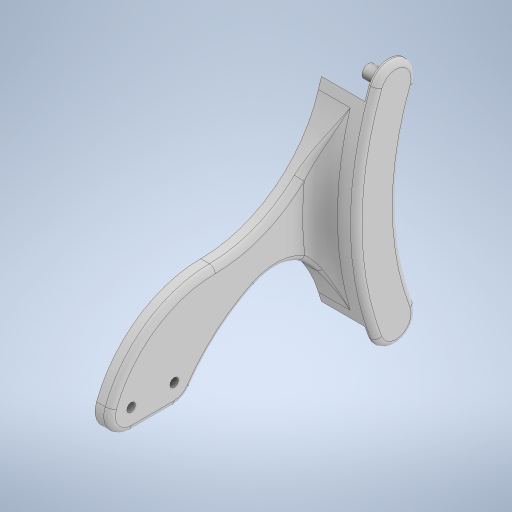
# Autodesk Inventor part: Soporte Selenoide
Saved by Autodesk Inventor 2023 (Build 270158000, 158)
## iProperties
Created: 2022-07-30
Part Number: Soporte Selenoide
Material: Genérico
Document SubType Name: Modeling
Designer: juand
Density: 1 g/cm^3
Appearance: Valor por defecto
Author: juand
Autodesk Inventor part; units mm, degrees
ref_plane "YZ Plane" through (0, 0, 0) normal (1, 0, 0) x (0, 1, 0)
ref_plane "XZ Plane" through (0, 0, 0) normal (0, 1, 0) x (-1, 0, 0)
ref_plane "XY Plane" through (0, 0, 0) normal (0, 0, 1) x (1, 0, 0)
sketch "Boceto1" plane through (0, 0, 0) normal (1, 0, 0) x (0, 1, 0)
  line L0 (0, 0) -> (-85, 0) construction
  line L1 (-85, 0) -> (-85, -100) construction
  line L2 (-85, -100) -> (0, -100) construction
  line L3 (0, -100) -> (0, 0) construction
  circle A0 centre (-7.25, -7.25) radius 2.25
  circle A1 centre (-77.75, -7.25) radius 2.25
  arc A2 (-9.8358, -14.0232) -> (-7.25, 0) centre (-7.25, -7.25) ccw
  arc A3 (-77.75, 0) -> (-75.1642, -14.0232) centre (-77.75, -7.25) ccw
  arc A4 (-9.8358, -14.0232) -> (-75.1642, -14.0232) centre (-42.5, -99.5817) ccw
  arc A5 (0, -2.3856) -> (-85, -2.3856) centre (-42.5, -99.5817) ccw
  line L4 (-8.7858, 1) -> (-76.2142, 1)
  line L5 (-65, 23) -> (-75, 23) construction
  line L6 (-75, 23) -> (-75, 13) construction
  line L7 (-75, 13) -> (-65, 13) construction
  line L8 (-65, 13) -> (-65, 23) construction
  circle A6 centre (-70, 57) radius 1.5
  circle A7 centre (-70, 71.9) radius 1.5
  arc A8 (-72.8434, 2.0677) -> (-42.5, 42.792) centre (-85, 42.792) ccw
  arc A9 (-42.5, 42.792) -> (-12.1566, 2.0677) centre (0, 42.792) ccw
  arc A10 (-67.3446, 78.8607) -> (-77.45, 71.9) centre (-70, 71.9) ccw
  arc A11 (-77.45, 57) -> (-74.1857, 50.837) centre (-70, 57) ccw
  line L9 (-77.45, 71.9) -> (-77.45, 57)
  arc A12 (-50.3466, 0) -> (-74.1857, 50.837) centre (-105.0869, 5.3385) ccw
  arc A13 (-42.5, 42.792) -> (-67.3446, 78.8607) centre (-81.1041, 42.792) ccw
  point P0 (-42.5, -8)
  point P1 (-42.5, 0)
  point P2 (-4.6642, -0.4768)
  point P3 (-80.3358, -0.4768)
  point P4 (-62.55, 57)
  point P5 (-51.3118, 16.8815)
  dimension "d0" = 100
  dimension "d1" = 85
  dimension "d2" = 70.5
  dimension "d3" = 7.25
  dimension "d4" = 7.25
  dimension "d5" = 14.9
  dimension "d6" = 15
  dimension "d7" = 157
  dimension "d8" = 4.5
  dimension "d11" = 8
  dimension "d14" = 1
  dimension "d17" = 10
  dimension "d18" = 10
  dimension "d19" = 23
  dimension "d20" = 10
  dimension "d22" = 3
  dimension "d23" = 110
  constraints: 26 point on circle, 20 end point, 14 centre point, 14 tangent, 8 coincident, 7 point on line, 5 parallel, 4 equal radius, 4 horizontal alignment, 2 horizontal, 2 perpendicular, 2 vertical alignment, 1 concentric, 1 midpoint
  measures "d0" distance of L2.end L0.start
  measures "d1" distance of L1.end L2.end
  measures "d2" distance of point (-77.75, -7.25) point (-7.25, -7.25)
  measures "d3" distance from line of L1 point (-77.75, -7.25)
  measures "d4" distance from line of L0 point (-77.75, -7.25)
  measures "d5" distance of point (-70, 57) point (-70, 71.9)
  measures "d6" distance from line of L1 point (-70, 57)
  measures "d7" distance from line of L2 point (-70, 57)
  measures "d8" diameter of A0
  measures "d11" distance of point (-42.5, -8) point (-42.5, 0)
  measures "d14" distance between parallel lines of L4 L0
  measures "d17" distance of L7.end L5.start
  measures "d18" distance of L6.end L7.end
  measures "d19" distance between parallel lines of L0 L5
  measures "d20" distance between parallel lines of L1 L6
  measures "d22" diameter of A6
  measures "d23" diameter of A12
extrude "Extrusión1" add sketch "Boceto1" against normal blind 7 contours A0 | A1
extrude "Extrusión2" add sketch "Boceto1" along normal blind 2.5 contours A0 | A1 | A4 A3 A5 L4 A2 | L4 A12 A5 | L4 A5 A12
extrude "Extrusión4" add sketch "Boceto1" against normal blind 15 contours L4 A12 A5 | A5 A12 A8 A9 | L4 A5 A12 | A5 A8 A12 | A8 A12 A11 L9 A10 A13
extrude "Extrusión5" cut sketch "Boceto1" against normal blind 10 contours A5 A12 A8 A9 | A5 A8 A12 | A8 A12 A11 L9 A10 A13
fillet "Empalme de cara1" radius 17 1 edges at (-12.5, -51.3118, 16.8815)
fillet "Empalme de cara2" radius 6 1 edges at (-10, -42.5, 6.5)
fillet "Empalme1" radius 2 14 edges at (2.5, -84.5232, -9.8358) (2.5, -42.5, -8) (2.5, -0.4768, -9.8358) (2.5, -42.5, 6.5) (-10, -63.3324, 41.1374) (-10, -76.5835, 53.513) (-10, -77.45, 64.45) (-10, -74.2261, 78.0353) (-10, -49.3122, 64.6907) (-10, -38.9659, 25.8241) (-7.8605, -20.6979, 5.6726) (-12.5, -61.2671, 7.5358) (-6.7049, -66.9908, 4.2963) (-10, -54.3649, 17.1449)
